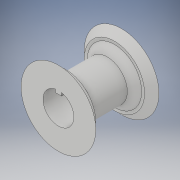
# Autodesk Inventor part: spool
Saved by Autodesk Inventor 2017 (Build 210142000, 142)
## iProperties
Created: 2018-02-17
Part Number: spool
Material: Generic
Document SubType Name: Modeling
Designer: Delta
Density: 1 g/cm^3
Appearance: Default
Author: Delta
Autodesk Inventor part; units mm, degrees
ref_plane "YZ Plane" through (0, 0, 0) normal (1, 0, 0) x (0, 1, 0)
ref_plane "XZ Plane" through (0, 0, 0) normal (0, 1, 0) x (-1, 0, 0)
ref_plane "XY Plane" through (0, 0, 0) normal (0, 0, 1) x (1, 0, 0)
sketch "Sketch1" plane through (0, 0, 0) normal (0, 0, 1) x (1, 0, 0)
  circle A0 centre (0, 0) radius 6.604
  circle A1 centre (0, 0) radius 16.51
  dimension "d0" = 13.208
  dimension "d1" = 33.02
  constraints: 2 centre point, 2 coincident
  measures "d0" diameter of A0
  measures "d1" diameter of A1
extrude "Extrusion1" add sketch "Sketch1" along normal blind 6.35
sketch "Sketch2" plane through (0, 0, 6.35) normal (0, 0, 1) x (1, 0, 0)
  circle A0 centre (0, 0) radius 6.604
  circle A1 centre (0, 0) radius 12.7
  dimension "d4" = 25.4
  constraints: 2 centre point, 2 coincident
  measures "d4" diameter of A1
extrude "Extrusion2" add sketch "Sketch2" along normal blind 15.24
sketch "Sketch3" plane through (0, 0, 21.59) normal (0, 0, 1) x (1, 0, 0)
  circle A0 centre (0, 0) radius 12.7
  circle A1 centre (0, 0) radius 16.51
  circle A2 centre (0, 0) radius 6.604
  dimension "d7" = 25.4
  dimension "d8" = 33.02
  dimension "d9" = 13.208
  constraints: 3 centre point, 3 coincident
  measures "d7" diameter of A0
  measures "d8" diameter of A1
  measures "d9" diameter of A2
extrude "Extrusion3" add sketch "Sketch3" along normal blind 6.35 contours A0 | A1
sketch "Sketch4" plane through (0, 0, 27.94) normal (0, 0, 1) x (1, 0, 0)
  circle A0 centre (0, 0) radius 6.604 projected
  line L0 (1.3879, 6.604) -> (-1.3553, 6.604)
  line L1 (-1.3553, 6.604) -> (-1.3553, 5.334)
  line L2 (-1.3553, 5.334) -> (1.3879, 5.334)
  line L3 (1.3879, 5.334) -> (1.3879, 6.604)
  point P0 (-2.9121, 5.9273)
  point P1 (-1.3626, 6.604)
  dimension "d12" = 2.7432
  dimension "d13" = 1.27
  constraints: 8 end point, 2 parallel, 1 horizontal, 1 perpendicular, 2 other
  measures "d12" distance of L2.end L1.end
  measures "d13" distance of L1.end L0.end
extrude "Extrusion4" add sketch "Sketch4" against normal blind 27.94 contours L3 L2 L1 A0 | A0 L0 L3 | L1 L0 A0 picked at (0.0109, 5.7573)
sketch "Sketch5" plane through (0, 0, 21.59) normal (0, 0, -1) x (-1, 0, 0)
  arc A0 (-1.3879, 6.4565) -> (1.3553, 6.4634) centre (0, 0) ccw projected
  circle A1 centre (0, 0) radius 12.7
  circle A2 centre (0, 0) radius 16.1987
  circle A3 centre (0, 0) radius 16.51
  dimension "d16" = 33.02
  constraints: 3 centre point, 3 coincident
  measures "d16" diameter of A3
extrude "Extrusion5" cut sketch "Sketch5" against normal blind 3.175 contours A2 | A3
sketch "Sketch6" plane through (0, 0, 6.35) normal (0, 0, 1) x (1, 0, 0)
  circle A0 centre (0, 0) radius 12.7
  circle A1 centre (0, 0) radius 16.51
  dimension "d19" = 25.4
  dimension "d20" = 33.02
  constraints: 2 centre point, 2 coincident
  measures "d19" diameter of A0
  measures "d20" diameter of A1
extrude "Extrusion6" cut sketch "Sketch6" against normal blind 3.175
sketch "Sketch7" plane through (0, 0, 3.175) normal (0, 0, 1) x (1, 0, 0)
  circle A0 centre (0, 0) radius 8.89
  circle A1 centre (0, 0) radius 12.7
  dimension "d23" = 17.78
  dimension "d24" = 25.4
  constraints: 2 centre point, 2 coincident
  measures "d23" diameter of A0
  measures "d24" diameter of A1
extrude "Extrusion7" cut sketch "Sketch7" along normal blind 21.59
chamfer "Chamfer1" distance 3.175 angle 45 4 edges at (-8.89, 0, 3.175) (-16.51, 0, 3.175) (-8.89, 0, 24.765) (-16.51, 0, 24.765)
sketch "Sketch8" plane through (0, 0, 27.94) normal (0, 0, 1) x (1, 0, 0)
  circle A0 centre (0, 0) radius 6.8262
  line L0 (-1.3553, 5.334) -> (-1.3553, 6.4634) projected
  line L1 (-1.3553, 6.6903) -> (-1.3553, 5.334)
  line L2 (1.3879, 6.4565) -> (1.3879, 5.334) projected
  line L3 (-1.3553, 5.334) -> (1.3879, 5.334)
  line L4 (1.3879, 5.334) -> (1.3879, 6.6837)
  dimension "d30" = 13.6525
  constraints: 6 end point, 2 perpendicular, 2 point on circle, 1 centre point, 1 coincident, 1 collinear
  measures "d30" diameter of A0
extrude "Extrusion8" cut sketch "Sketch8" against normal blind 50.8 contours A0 L1 L0 L3 L2 L4 picked at (-0.1975, 1.2902)
body "Solid1"
